Autodesk Fusion 360 part; units mm, degrees
note: some values were not read from the file. Set by a fixed rule: which sketch regions a step uses.
(part 2 of 2)
extrude "Extrude2'''''" cut sketch "End leg - wave" against normal blind 2.54 contours A3 A9 L22 A21 bodies 21 in component "End leg - left (1) (1)"
extrude "Extrude1''''''''''''''''''''" add sketch "Inner leg" along normal blind 18.542 separate body contours L0 L1 L2 A0 A1 L4 L5 A2 L6 A3 L7 L9 L10 L12 A4 A5 L13 L14 L16 A6 A7 L18 L19 L20 L22 L23 L24 A8 A9 A10 A11 L34 L35 L36 L37 L38 L39 L40 A23 A24 L43 L44 L45 A25 makes body 22 in component "Inner leg - right -- middle (1)"
extrude "Extrude1'''''''''''''''''''''" add sketch "Inner leg" along normal blind 18.542 separate body contours L0 L1 L2 A0 A1 L4 L5 A2 L6 A3 L7 L9 L10 L12 A4 A5 L13 L14 L16 A6 A7 L18 L19 L20 L22 L23 L24 A8 A9 A10 A11 L34 L35 L36 L37 L38 L39 L40 A23 A24 L43 L44 L45 A25 makes body 23 in component "Inner leg - right -- left (1)"
extrude "Extrude1''''''''''''''''''''''" add sketch "Inner leg" along normal blind 18.542 separate body contours L0 L1 L2 A0 A1 L4 L5 A2 L6 A3 L7 L9 L10 L12 A4 A5 L13 L14 L16 A6 A7 L18 L19 L20 L22 L23 L24 A8 A9 A10 A11 L34 L35 L36 L37 L38 L39 L40 A23 A24 L43 L44 L45 A25 makes body 24 in component "Inner leg - left -- right (1)"
extrude "Extrude1'''''''''''''''''''''''" add sketch "Inner end leg" along normal blind 18.542 separate body contours A0 L1 L2 L3 A1 L4 A2 A3 A4 A5 L6 L7 L8 L9 A6 A7 L10 L12 A8 L14 A9 L15 L17 L19 L20 L21 L22 A18 L31 L32 L33 L34 L35 L36 L38 L39 L40 L42 A19 A20 makes body 25 in component "Inner leg end (1)"
extrude "Extrude1''''''''''''''''''''''''" add sketch "Inner leg" along normal blind 18.542 separate body contours L0 L1 L2 A0 A1 L4 L5 A2 L6 A3 L7 L9 L10 L12 A4 A5 L13 L14 L16 A6 A7 L18 L19 L20 L22 L23 L24 A8 A9 A10 A11 L34 L35 L36 L37 L38 L39 L40 A23 A24 L43 L44 L45 A25 makes body 26 in component "Inner leg - left -- left (1)"
extrude "Extrude1'''''''''''''''''''''''''" add sketch "Surface" against normal blind 18.542 separate body makes body 27 in component "Surface - right (1)"
extrude "Extrude2''''''" cut sketch "Surface" against normal blind 6.1807 contours L1 L3 L13 L15 | L1 L3 L10 L12 | L1 L3 L7 L9 | L1 L3 A0 L4 L6 bodies 27 in component "Surface - right (1)"
extrude "Extrude1''''''''''''''''''''''''''" add sketch "Spine - long" along normal blind 18.542 separate body contours L0 L3 L4 L5 L7 L8 L9 L11 L12 L13 L14 L15 L16 L21 A0 A1 A2 L27 A6 A7 A8 A9 A10 A11 A12 L30 L31 L32 L33 L34 L39 | L22 L26 L27 L40 | L18 L23 A3 A4 L25 L26 L38 L44 | L19 L24 L25 L46 | L1 L20 A5 L24 A13 L36 L45 | L20 A5 picked at (-72.5108, 47.7756) makes body 28 in component "Long spine (1) (1)"
extrude "Extrude1'''''''''''''''''''''''''''" add sketch "Spine - long" along normal blind 18.542 separate body contours L0 L3 L4 L5 L7 L8 L9 L11 L12 L13 L14 L15 L16 L21 A0 A1 A2 L27 A6 A7 A8 A9 A10 A11 A12 L30 L31 L32 L33 L34 L39 | L22 L26 L27 L40 | L18 L23 A3 A4 L25 L26 L38 L44 | L19 L24 L25 L46 | L1 L20 A5 L24 A13 L36 L45 | L20 A5 picked at (-72.5108, 47.7756) makes body 29 in component "Long spine (1) (2)"
extrude "Extrude1''''''''''''''''''''''''''''" add sketch "Surface" along normal blind 18.542 separate body makes body 30 in component "Surface - left (1)"
extrude "Extrude2'''''''" cut sketch "Surface" along normal blind 6.1807 contours L1 L3 L13 L15 | L1 L3 L10 L12 | L1 L3 L7 L9 | L1 L3 A0 L4 L6 bodies 30 in component "Surface - left (1)"
extrude "Extrude1'''''''''''''''''''''''''''''" add sketch "Spine - short" along normal blind 18.542 separate body contours L0 L1 L3 L4 L5 L6 L7 L8 L10 L11 L12 L14 L15 L16 A0 A1 A2 A3 A4 A5 A6 A7 L17 L18 L19 L20 L21 L22 A8 A9 A10 A11 A12 A13 L23 L24 L26 L27 L29 L30 L32 L33 makes body 31 in component "Short spine (1)"
extrude "Extrude1''''''''''''''''''''''''''''''" add sketch "Spine - short" along normal blind 18.542 separate body contours L0 L1 L3 L4 L5 L6 L7 L8 L10 L11 L12 L14 L15 L16 A0 A1 A2 A3 A4 A5 A6 A7 L17 L18 L19 L20 L21 L22 A8 A9 A10 A11 A12 A13 L23 L24 L26 L27 L29 L30 L32 L33 makes body 32 in component "Short spine (2)"
extrude "Extrude1'''''''''''''''''''''''''''''''" add sketch "Shelf" along normal blind 18.542 separate body contours L0 L1 L2 L3 L4 L5 A0 A1 A2 A3 L8 L9 L10 L12 L13 L14 L15 L16 L17 A4 A5 A6 A7 A8 A9 A10 A11 L18 L19 L20 L22 L23 makes body 33 in component "Shelf - left -- upper (1)"
copy_body "CopyPasteBodies1'" bodies 15 makes body 34 in component "Shelf - left -- lower (1)"
extrude "Extrude1''''''''''''''''''''''''''''''''" add sketch "Shelf" along normal blind 18.542 separate body contours L0 L1 L2 L3 L4 L5 A0 A1 A2 A3 L8 L9 L10 L12 L13 L14 L15 L16 L17 A4 A5 A6 A7 A8 A9 A10 A11 L18 L19 L20 L22 L23 makes body 35 in component "Shelf - right -- lower (1)"
extrude "Extrude1'''''''''''''''''''''''''''''''''" add sketch "Shelf" along normal blind 18.542 separate body contours L0 L1 L2 L3 L4 L5 A0 A1 A2 A3 L8 L9 L10 L12 L13 L14 L15 L16 L17 A4 A5 A6 A7 A8 A9 A10 A11 L18 L19 L20 L22 L23 makes body 36 in component "Shelf - right -- upper (1)"
extrude "Extrude1''''''''''''''''''''''''''''''''''" add sketch "Shelf" along normal blind 18.542 separate body contours L0 L1 L2 L3 L4 L5 A0 A1 A2 A3 L8 L9 L10 L12 L13 L14 L15 L16 L17 A4 A5 A6 A7 A8 A9 A10 A11 L18 L19 L20 L22 L23 makes body 37 in component "Shelf"
sketch "Stock - shelf jig" plane through (0, 0, 0) normal (0, 1, 0) x (1, 0, 0)
  line L0 (0, 0) -> (873.125, 0)
  line L1 (873.125, 0) -> (873.125, 254)
  line L2 (873.125, 254) -> (0, 254)
  line L3 (0, 254) -> (0, 0)
  dimension "d3885" = 873.125
  dimension "d3886" = 254
  measures "d3885" distance of L0.start L0.end
  measures "d3886" distance of L0.start L2.end
extrude "Extrude1'''''''''''''''''''''''''''''''''''" add sketch "Stock - shelf jig" along normal blind 18.542 separate body makes body 38 in component "Stock - shelf"
sketch "Stock - spine (long) jig" plane through (0, 0, 0) normal (0, 1, 0) x (1, 0, 0)
  line L0 (0, 0) -> (1168.4, 0)
  line L1 (1168.4, 0) -> (1168.4, 101.6)
  line L2 (1168.4, 101.6) -> (0, 101.6)
  line L3 (0, 101.6) -> (0, 0)
  line L4 (787.4, 0) -> (787.4, 101.6)
  dimension "d3905" = 101.6
  dimension "d3906" = 1168.4
  dimension "d3938" = 787.4
  measures "d3905" distance of L0.start L2.end
  measures "d3906" distance of L0.start L0.end
  measures "d3938" distance of L3 L4
extrude "Extrude1''''''''''''''''''''''''''''''''''''" add sketch "Stock - spine (long) jig" along normal blind 18.542 separate body contours L0 L2 L3 L4 makes body 39 in component "Stock - spine (long) - bottom"
extrude "Extrude1'''''''''''''''''''''''''''''''''''''" add sketch "Stock - spine (long) jig" along normal blind 18.542 separate body makes body 40 in component "Stock - spine (long) - top"
extrude "Extrude1''''''''''''''''''''''''''''''''''''''" add sketch "Spine - long" along normal blind 18.542 separate body contours L0 L3 L4 L5 L7 L8 L9 L11 L12 L13 L14 L15 L16 L21 A0 A1 A2 L27 A6 A7 A8 A9 A10 A11 A12 L30 L31 L32 L33 L34 L39 | L22 L26 L27 L40 | L18 L23 A3 A4 L25 L26 L38 L44 | L19 L24 L25 L46 | L1 L20 A5 L24 A13 L36 L45 | L20 A5 picked at (-72.5108, 47.7756) makes body 41 in component "Spine (long) - top"
extrude "Extrude1'''''''''''''''''''''''''''''''''''''''" add sketch "Spine - long" along normal blind 18.542 separate body contours L0 L3 L4 L5 L7 L8 L9 L11 L12 L13 L14 L15 L16 L21 A0 A1 A2 L27 A6 A7 A8 A9 A10 A11 A12 L30 L31 L32 L33 L34 L39 | L22 L26 L27 L40 | L18 L23 A3 A4 L25 L26 L38 L44 | L19 L24 L25 L46 | L1 L20 A5 L24 A13 L36 L45 | L20 A5 picked at (-72.5108, 47.7756) makes body 42 in component "Spine (long) - bottom"
sketch "Stock - spine (short) jig" plane through (0, 0, 0) normal (0, 1, 0) x (1, 0, 0)
  line L0 (0, 0) -> (914.4, 0)
  line L1 (914.4, 0) -> (914.4, 101.6)
  line L2 (914.4, 101.6) -> (0, 101.6)
  line L3 (0, 101.6) -> (0, 0)
  dimension "d3943" = 101.6
  dimension "d3944" = 914.4
  measures "d3943" distance of L0.start L2.end
  measures "d3944" distance of L0.start L0.end
extrude "Extrude1''''''''''''''''''''''''''''''''''''''''" add sketch "Stock - spine (short) jig" along normal blind 18.542 separate body makes body 43 in component "Stock - spine (short)"
extrude "Extrude1'''''''''''''''''''''''''''''''''''''''''" add sketch "Spine - short" along normal blind 18.542 separate body contours L0 L1 L3 L4 L5 L6 L7 L8 L10 L11 L12 L14 L15 L16 A0 A1 A2 A3 A4 A5 A6 A7 L17 L18 L19 L20 L21 L22 A8 A9 A10 A11 A12 A13 L23 L24 L26 L27 L29 L30 L32 L33 makes body 44 in component "Spine (short) - top"
extrude "Extrude1''''''''''''''''''''''''''''''''''''''''''" add sketch "Spine - short" along normal blind 18.542 separate body contours L0 L1 L3 L4 L5 L6 L7 L8 L10 L11 L12 L14 L15 L16 A0 A1 A2 A3 A4 A5 A6 A7 L17 L18 L19 L20 L21 L22 A8 A9 A10 A11 A12 A13 L23 L24 L26 L27 L29 L30 L32 L33 makes body 45 in component "Spine (short) - bottom"
extrude "Extrude1'''''''''''''''''''''''''''''''''''''''''''" add sketch "Surface" against normal blind 18.542 separate body makes body 46 in component "Surface for radius operation"
extrude "Extrude2''''''''" cut sketch "Surface" against normal blind 6.1807 contours L1 L3 L13 L15 | L1 L3 L10 L12 | L1 L3 L7 L9 | L1 L3 A0 L4 L6 bodies 46 in component "Surface for radius operation"
sketch "Stock - surface radius jig" plane through (0, 0, 0) normal (0, 1, 0) x (1, 0, 0)
  line L0 (0, 0) -> (76.2, 0)
  line L1 (76.2, 0) -> (76.2, 762)
  line L2 (76.2, 762) -> (0, 762)
  line L3 (0, 762) -> (0, 0)
  dimension "d4039" = 762
  dimension "d4040" = 76.2
  measures "d4039" distance of L0.start L2.end
  measures "d4040" distance of L0.start L0.end
extrude "Extrude1''''''''''''''''''''''''''''''''''''''''''''" add sketch "Stock - surface radius jig" along normal blind 18.542 separate body makes body 47 in component "Stock - surface radius"
extrude "Extrude1'''''''''''''''''''''''''''''''''''''''''''''" add sketch "Surface" against normal blind 18.542 separate body makes body 48 in component "Surface for slot operation"
extrude "Extrude2'''''''''" cut sketch "Surface" against normal blind 6.1807 contours L1 L3 L13 L15 | L1 L3 L10 L12 | L1 L3 L7 L9 | L1 L3 A0 L4 L6 bodies 48 in component "Surface for slot operation"
component "Assembled" placed x (1, 0, 0) y (0, 1, 0) z (0, 0, 1) at (0, 0, 0)
component "Fabrication" placed x (1, 0, 0) y (0, 1, 0) z (0, 0, 1) at (0, 0, 0)
component "Surface - left" placed x (0, 0, -1) y (0, 1, 0) z (1, 0, 0) at (2582.0041, 744.1354, 574.929) in component "Surfaces"
component "Surface - right" placed x (-1, 0, 0) y (0, -1, 0) z (0, 0, 1) at (1820.037, 744.1354, 571.4671) in component "Surfaces"
component "Inner leg - left -- left" placed x (1, 0, 0) y (0, 1, 0) z (0, 0, 1) at (2582.1218, 0.6388, -723.392) in component "Left side"
component "Inner leg - left -- right" placed x (1, 0, 0) y (0, 1, 0) z (0, 0, 1) at (2582.1218, 0.6388, -183.642) in component "Left side"
component "Inner leg end" placed x (1, 0, 0) y (0, 1, 0) z (0, 0, 1) at (2582.037, 0.6388, 356.108) in component "Left side"
component "Inner leg - right -- right" placed x (0, 0, 1) y (0, 1, 0) z (-1, 0, 0) at (540.258, 0, 571.5) in component "Right side"
component "Inner leg - right -- middle" placed x (0, 0, 1) y (0, 1, 0) z (-1, 0, 0) at (1080.008, 0, 571.5) in component "Right side"
component "Inner leg - right -- left" placed x (0, 0, 1) y (0, 1, 0) z (-1, 0, 0) at (1619.758, 0, 571.5) in component "Right side"
component "Left side" placed x (1, 0, 0) y (0, 1, 0) z (0, 0, 1) at (0, 0, 0) in component "Inner legs"
component "Right side" placed x (1, 0, 0) y (0, 1, 0) z (0, 0, 1) at (0, 0, 0) in component "Inner legs"
component "Shelves -- left" placed x (1, 0, 0) y (0, 1, 0) z (0, 0, 1) at (0, 0, 0) in component "Shelves"
component "Shelves -- right" placed x (1, 0, 0) y (0, 1, 0) z (0, 0, 1) at (0, 0, 0) in component "Shelves"
component "Shelf - left -- upper" placed x (1, 0, 0) y (0, 1, 0) z (0, 0, 1) at (2328.037, 420.3954, 428.879) in component "Shelves -- left"
component "Shelf - left -- lower" placed x (1, 0, 0) y (0, 1, 0) z (0, 0, 1) at (2328.037, 115.5954, 428.879) in component "Shelves -- left"
component "Long spines" placed x (1, 0, 0) y (0, 1, 0) z (0, 0, 1) at (0, 0, 0) in component "Spines"
component "Short spines" placed x (1, 0, 0) y (0, 1, 0) z (0, 0, 1) at (0, 0, 0) in component "Spines"
component "Long spine (1)" placed x (1, 0, 0) y (0, 1, 0) z (0, 0, 1) at (2366.137, 641.731, 98.679) in component "Long spines"
component "Long spine (1)" placed x (1, 0, 0) y (0, 1, 0) z (0, 0, 1) at (2366.137, 642.4968, 263.779) in component "Long spines"
component "Short spine" placed x (1, 0, 0) y (0, 1, 0) z (0, 0, 1) at (2109.216, 642.4968, 511.429) in component "Short spines"
component "Short spine" placed x (1, 0, 0) y (0, 1, 0) z (0, 0, 1) at (2274.316, 642.4968, 511.429) in component "Short spines"
component "End leg - right (1)" placed x (1, 0, 0) y (0, 1, 0) z (0, 0, 1) at (-18.034, 0, 0) in component "End legs"
component "End leg - left (1)" placed x (0, 0, -1) y (0, 1, 0) z (1, 0, 0) at (2010.537, 0, -1263.142) in component "End legs"
component "Surfaces" placed x (1, 0, 0) y (0, 1, 0) z (0, 0, 1) at (0, 0, 0) in component "Assembled"
component "Inner legs" placed x (1, 0, 0) y (0, 1, 0) z (0, 0, 1) at (0, 0, 0) in component "Assembled"
component "Shelves" placed x (1, 0, 0) y (0, 1, 0) z (0, 0, 1) at (0, 0, 0) in component "Assembled"
component "Spines" placed x (1, 0, 0) y (0, 1, 0) z (0, 0, 1) at (0, 0, 0) in component "Assembled"
component "End legs" placed x (1, 0, 0) y (0, 1, 0) z (0, 0, 1) at (0, 0, 0) in component "Assembled"
component "Stock - 4x8'" placed x (1, 0, 0) y (0, 1, 0) z (0, 0, 1) at (0, 0, 0) in component "Fabrication"
component "Stock - 4x4'" placed x (1, 0, 0) y (0, 1, 0) z (0, 0, 1) at (0, 0, 0) in component "Fabrication"
component "Sheet 1 - end leg (right) + inner leg x1" placed x (1, 0, 0) y (0, 1, 0) z (0, 0, 1) at (0, 0, 0) in component "Fabrication"
component "Sheet 2 - end leg (left) + inner leg x1" placed x (1, 0, 0) y (0, 1, 0) z (0, 0, 1) at (0, 0, 0) in component "Fabrication"
component "Sheet 3 - inner leg x2" placed x (1, 0, 0) y (0, 1, 0) z (0, 0, 1) at (0, 0, 0) in component "Fabrication"
component "Sheet 4 - inner end leg + inner leg x1" placed x (1, 0, 0) y (0, 1, 0) z (0, 0, 1) at (0, 0, 0) in component "Fabrication"
component "Sheet 5 - surface (right) + long spines" placed x (1, 0, 0) y (0, 1, 0) z (0, 0, 1) at (0, 0, 0) in component "Fabrication"
component "Sheet 6 - surface (left) + short spines" placed x (1, 0, 0) y (0, 1, 0) z (0, 0, 1) at (0, 0, 0) in component "Fabrication"
component "Sheet 7 - shelves" placed x (1, 0, 0) y (0, 1, 0) z (0, 0, 1) at (0, 0, 0) in component "Fabrication"
component "Jig - shelf" placed x (1, 0, 0) y (0, 1, 0) z (0, 0, 1) at (0, 0, 0) in component "Fabrication"
component "Jigs - long spine" placed x (1, 0, 0) y (0, 1, 0) z (0, 0, 1) at (0, 0, 0) in component "Fabrication"
component "Jigs - short spine" placed x (1, 0, 0) y (0, 1, 0) z (0, 0, 1) at (0, 0, 0) in component "Fabrication"
component "Jigs - surface radius and slot" placed x (1, 0, 0) y (0, 1, 0) z (0, 0, 1) at (0, 0, 0) in component "Fabrication"
component "Shelf - right -- lower" placed x (0, 0, 1) y (0, 1, 0) z (-1, 0, 0) at (-72.263, 115.5954, 317.5) in component "Shelves -- right"
component "Shelf - right -- upper" placed x (0, 0, 1) y (0, 1, 0) z (-1, 0, 0) at (-72.263, 420.3954, 317.5) in component "Shelves -- right"
component "End leg - right (1) (1)" placed x (0, -1, 0) y (1, 0, 0) z (0, 0, 1) at (408.533, 18.542, 520.0921) in component "Sheet 1 - end leg (right) + inner leg x1"
component "Inner leg - right -- right (1)" placed x (-1, 0, 0) y (0, 0, -1) z (0, -1, 0) at (78.8, 18.542, 990.0892) in component "Sheet 1 - end leg (right) + inner leg x1"
component "End leg - left (1) (1)" placed x (0, 1, 0) y (0, 0, 1) z (1, 0, 0) at (296.1006, 18.542, 127.0302) in component "Sheet 2 - end leg (left) + inner leg x1"
component "Inner leg - right -- middle (1)" placed x (-1, 0, 0) y (0, 0, -1) z (0, -1, 0) at (454.1371, 18.542, 1099.058) in component "Sheet 2 - end leg (left) + inner leg x1"
component "Inner leg - right -- left (1)" placed x (-1, 0, 0) y (0, 0, -1) z (0, -1, 0) at (454.1371, 18.542, 1099.058) in component "Sheet 3 - inner leg x2"
component "Inner leg - left -- right (1)" placed x (1, 0, 0) y (0, 0, 1) z (0, -1, 0) at (765.0629, 18.542, 120.142) in component "Sheet 3 - inner leg x2"
component "Inner leg end (1)" placed x (0, 0, -1) y (1, 0, 0) z (0, -1, 0) at (107.442, 18.542, 274.1395) in component "Sheet 4 - inner end leg + inner leg x1"
component "Inner leg - left -- left (1)" placed x (1, 0, 0) y (0, 0, 1) z (0, -1, 0) at (765.0629, 18.542, 120.142) in component "Sheet 4 - inner end leg + inner leg x1"
component "Surface - right (1)" placed x (1, 0, 0) y (0, 1, 0) z (0, 0, 1) at (266.7, 18.542, 990.6) in component "Sheet 5 - surface (right) + long spines"
component "Long spine (1) (1)" placed x (1, 0, 0) y (0, 0, 1) z (0, -1, 0) at (2438.4, 18.542, 558.8) in component "Sheet 5 - surface (right) + long spines"
component "Long spine (1) (2)" placed x (1, 0, 0) y (0, 0, 1) z (0, -1, 0) at (2438.4, 18.542, 558.8) in component "Sheet 5 - surface (right) + long spines"
component "Surface - left (1)" placed x (1, 0, 0) y (0, -1, 0) z (0, 0, -1) at (266.7, 18.542, 228.6) in component "Sheet 6 - surface (left) + short spines"
component "Short spine (1)" placed x (0, 1, 0) y (0, 0, 1) z (1, 0, 0) at (2133.6, 0, 558.8) in component "Sheet 6 - surface (left) + short spines"
component "Short spine (2)" placed x (0, 1, 0) y (0, 0, 1) z (1, 0, 0) at (2133.6, 0, 558.8) in component "Sheet 6 - surface (left) + short spines"
component "Shelf - left -- upper (1)" placed x (0, 0, -1) y (0, -1, 0) z (-1, 0, 0) at (346.075, 18.542, 736.6) in component "Sheet 7 - shelves"
component "Shelf - left -- lower (1)" placed x (0, 0, -1) y (0, -1, 0) z (-1, 0, 0) at (346.075, 18.542, 736.6) in component "Sheet 7 - shelves"
component "Shelf - right -- lower (1)" placed x (0, 0, 1) y (0, -1, 0) z (1, 0, 0) at (2092.325, 18.542, 482.6) in component "Sheet 7 - shelves"
component "Shelf - right -- upper (1)" placed x (0, 0, 1) y (0, -1, 0) z (1, 0, 0) at (2092.325, 18.542, 482.6) in component "Sheet 7 - shelves"
component "Shelf" placed x (0, 0, 1) y (0, 1, 0) z (-1, 0, 0) at (-873.125, 0, -254) in component "Jig - shelf"
component "Stock - shelf" placed x (1, 0, 0) y (0, 1, 0) z (0, 0, 1) at (0, 0, 0) in component "Jig - shelf"
component "Stock - spine (long) - top" placed x (1, 0, 0) y (0, 1, 0) z (0, 0, 1) at (0, 0, 0) in component "Jigs - long spine"
component "Spine (long) - top" placed x (-1, 0, 0) y (0, 0, 1) z (0, 1, 0) at (-1270, 0, -101.6) in component "Jigs - long spine"
component "Spine (long) - bottom" placed x (1, 0, 0) y (0, 0, 1) z (0, -1, 0) at (787.4, 18.542, -101.6) in component "Jigs - long spine"
component "Stock - spine (long) - bottom" placed x (1, 0, 0) y (0, 1, 0) z (0, 0, 1) at (0, 0, 0) in component "Jigs - long spine"
component "Stock - spine (short)" placed x (1, 0, 0) y (0, 1, 0) z (0, 0, 1) at (0, 0, 0) in component "Jigs - short spine"
component "Spine (short) - top" placed x (0, 1, 0) y (0, 0, 1) z (1, 0, 0) at (914.4, 0, -101.6) in component "Jigs - short spine"
component "Spine (short) - bottom" placed x (0, -1, 0) y (0, 0, 1) z (-1, 0, 0) at (-914.4, 18.542, -101.6) in component "Jigs - short spine"
component "Surface for radius operation" placed x (1, 0, 0) y (0, 1, 0) z (0, 0, 1) at (-1828.8, 18.542, 0) in component "Jigs - surface radius and slot"
component "Stock - surface radius" placed x (1, 0, 0) y (0, 1, 0) z (0, 0, 1) at (0, 0, 0) in component "Jigs - surface radius and slot"
component "Surface for slot operation" placed x (1, 0, 0) y (0, 1, 0) z (0, 0, 1) at (-199.009, 18.542, 762) in component "Jigs - surface radius and slot"
equation "d2 = Depth"
equation "Depth = 30 in"
equation "Thickness_Surface = Thickness_Global"
equation "SegmentLength = 72 in"
equation "Thickness_Legs = Thickness_Global"
equation "Fit_Interference = ( 0.011 * 2 ) * 1 in"
equation "Fit_Clearance = 0.1 in"
equation "d25 = Bench_Height - Thickness_Surface"
equation "Bench_Height = 30 in"
equation "d27 = Depth * 0.75"
equation "Depth_Engrave = 0.1 in"
equation "d38 = d37"
equation "d41 = Thickness_Legs"
equation "Bolt_Diameter = 8 mm"
equation "d45 = 21.25 in"
equation "d46 = d45"
equation "d48 = d52 / 2"
equation "d49 = d48"
equation "d50 = d49"
equation "d52 = d2 / 2"
equation "d54 = d52"
equation "d55 = d54"
equation "d103 = Depth / 3"
equation "d41_1 = Thickness_Legs"
equation "d41_2 = Thickness_Legs"
equation "d41_2_1 = Thickness_Legs"
equation "d41_2_2 = Thickness_Legs"
equation "d121 = d2 / 2"
equation "d122 = d121"
equation "Lower_Shelf_Height = Bench_Height / 5 - Thickness_Legs"
equation "d129 = End_Mill_Diameter"
equation "End_Mill_Diameter = 0.25 in"
equation "d133 = Shelf_Support_Thickness + Fit_Clearance"
equation "d136 = Shelf_Support_Height / 2"
equation "d137 = Lower_Shelf_Height"
equation "d138 = d103 / 5"
equation "Shelf_Support_Height = 2.5 in"
equation "d151 = d136"
equation "d152 = d138"
equation "d153 = Upper_Shelf_Height"
equation "Upper_Shelf_Height = Bench_Height / 5 * 3 - Thickness_Legs"
equation "d162 = d171"
equation "d171 = Shelf_Support_Thickness + Fit_Clearance"
equation "d176 = d162"
equation "d182 = End_Mill_Diameter"
equation "d183 = End_Mill_Diameter"
equation "Shelf_Support_Thickness = Thickness_Global"
equation "d249 = Lower_Shelf_Height"
equation "Shelf_Support_Length = ( 4 * 12 ) * 1 in"
equation "d270 = d46"
equation "d277 = d270"
equation "d280 = d277 / 2"
equation "d283 = d50"
equation "d286 = d50"
equation "d289 = d286"
equation "Shelf_Depth = 10 in"
equation "d314 = Thickness_Shelf - Fit_Interference"
equation "d316 = End_Mill_Diameter"
equation "d317 = End_Mill_Diameter"
equation "Thickness_Shelf = Thickness_Legs"
equation "d320 = d314"
equation "d322 = End_Mill_Diameter"
equation "d323 = End_Mill_Diameter"
equation "d328 = Shelf_Depth / 2"
equation "d329 = End_Mill_Diameter"
equation "d330 = End_Mill_Diameter"
equation "d331 = Thickness_Shelf - Fit_Interference"
equation "d332 = Upper_Shelf_Height"
equation "d333 = d328"
equation "d334 = d331"
equation "d335 = End_Mill_Diameter"
equation "d336 = End_Mill_Diameter"
equation "d337 = Lower_Shelf_Height"
equation "d382 = Cable_Channel_Width"
equation "d385 = Cable_Channel_Width"
equation "Tab_Size = 2 in"
equation "d466 = Depth / 2 / 2"
equation "d493 = Shelf_Depth / 2"
equation "d494 = Thickness_Legs - Fit_Interference"
equation "d497 = d496"
equation "d498 = d499"
equation "d499 = d497"
equation "d500 = d493"
equation "d501 = d494"
equation "d503 = d501"
equation "d504 = d500"
equation "d505 = d502"
equation "d506 = d504"
equation "d507 = d503"
equation "d508 = d505"
equation "d509 = End_Mill_Diameter"
equation "d510 = End_Mill_Diameter"
equation "d511 = End_Mill_Diameter"
equation "d512 = End_Mill_Diameter"
equation "d513 = End_Mill_Diameter"
equation "d514 = End_Mill_Diameter"
equation "d515 = End_Mill_Diameter"
equation "d516 = End_Mill_Diameter"
equation "Spine_Height = 4 in"
equation "d772 = Thickness_Legs - Fit_Interference"
equation "d773 = Spine_Height / 2"
equation "d774 = d772"
equation "d775 = Spine_Height / 2"
equation "d776 = End_Mill_Diameter"
equation "d777 = End_Mill_Diameter"
equation "d778 = End_Mill_Diameter"
equation "d779 = End_Mill_Diameter"
equation "d781 = 13.00 in / 2"
equation "d782 = d781 / 2"
equation "d783 = d782"
equation "d834 = Spine_Height"
equation "d835 = Thickness_Legs"
equation "d839 = Thickness_Legs - Fit_Interference"
equation "d840 = Spine_Height / 2"
equation "d841 = d839"
equation "d842 = d840"
equation "d843 = d842"
equation "d844 = d841"
equation "d845 = d846"
equation "d848 = d844"
equation "d849 = d843"
equation "d850 = d853"
equation "d851 = d852"
equation "d852 = d849"
equation "d853 = d848"
equation "d854 = d845"
equation "d857 = End_Mill_Diameter"
equation "d858 = End_Mill_Diameter"
equation "d859 = End_Mill_Diameter"
equation "d860 = End_Mill_Diameter"
equation "d861 = End_Mill_Diameter"
equation "d862 = End_Mill_Diameter"
equation "d863 = End_Mill_Diameter"
equation "d864 = End_Mill_Diameter"
equation "d865 = End_Mill_Diameter"
equation "d866 = End_Mill_Diameter"
equation "d867 = End_Mill_Diameter"
equation "d868 = End_Mill_Diameter"
equation "d869 = Thickness_Legs - Fit_Interference"
equation "d870 = Spine_Height / 2"
equation "d871 = d869"
equation "d872 = d870"
equation "d875 = 13.00 in / 2"
equation "d876 = d875 / 2"
equation "d877 = d876"
equation "d878 = End_Mill_Diameter"
equation "d879 = End_Mill_Diameter"
equation "d880 = End_Mill_Diameter"
equation "d881 = End_Mill_Diameter"
equation "d906 = 6'-0\""
equation "d907 = Spine_Height"
equation "d908 = Thickness_Legs - Fit_Interference"
equation "d909 = Spine_Height / 2"
equation "d912 = d908"
equation "d913 = d909"
equation "d914 = d912"
equation "d915 = d913"
equation "d916 = d969"
equation "d917 = d970"
equation "d926 = Thickness_Legs"
equation "d928 = End_Mill_Diameter"
equation "d929 = End_Mill_Diameter"
equation "d930 = End_Mill_Diameter"
equation "d931 = End_Mill_Diameter"
equation "d932 = End_Mill_Diameter"
equation "d933 = End_Mill_Diameter"
equation "d934 = End_Mill_Diameter"
equation "d935 = End_Mill_Diameter"
equation "d969 = d1382"
equation "d970 = d972"
equation "d972 = d915"
equation "d973 = End_Mill_Diameter"
equation "d974 = End_Mill_Diameter"
equation "d975 = End_Mill_Diameter"
equation "d976 = End_Mill_Diameter"
equation "d977 = 4 in - Thickness_Legs / 2"
equation "d982 = Spine_Height / 2"
equation "d983 = Spine_Height / 2"
equation "d984 = Spine_Height / 2"
equation "d985 = Spine_Height / 2"
equation "d987 = Shelf_Depth / 2"
equation "d1017 = Thickness_Shelf - Fit_Interference"
equation "d1019 = End_Mill_Diameter"
equation "d1020 = End_Mill_Diameter"
equation "d1021 = d1017"
equation "d1023 = End_Mill_Diameter"
equation "d1024 = End_Mill_Diameter"
equation "d1025 = d314 / 2"
equation "d1026 = d320 / 2"
equation "d1033 = Thickness_Legs - Fit_Interference"
equation "d1034 = Spine_Height / 2"
equation "d1036 = d1034"
equation "d1037 = End_Mill_Diameter"
equation "d1038 = End_Mill_Diameter"
equation "d1039 = End_Mill_Diameter"
equation "d1040 = End_Mill_Diameter"
equation "d1042 = d781 / 2"
equation "d1043 = d782"
equation "d1062 = Lower_Shelf_Height"
equation "d1063 = Upper_Shelf_Height"
equation "d1064 = Thickness_Legs"
equation "d1107 = d1106"
equation "d1108 = d1105"
equation "d1109 = d1104"
equation "d1110 = d1109"
equation "d1382 = d914"
equation "d2574 = d2571"
equation "d2577 = d2571"
equation "d2653 = 3 in"
equation "d2663 = d2653"
equation "d2674 = d2663"
equation "Thickness_Global = 0.73 in"
equation "d2750 = End_Mill_Diameter"
equation "d2751 = End_Mill_Diameter"
equation "d2754 = Thickness_Global"
equation "Leg_Spacing = 21.25 in"
equation "d2962 = Shelf_Depth / 2"
equation "d2964 = d1250"
equation "d2965 = Shelf_Depth / 2"
equation "d2969 = Thickness_Surface / 3"
equation "d2970 = Thickness_Surface / 3"
equation "d2972 = Bench_Height - Thickness_Surface + Thickness_Surface / 3"
equation "d2974 = Thickness_Legs - Fit_Interference"
equation "d2975 = d2974"
equation "d2976 = d1062"
equation "Cable_Channel_Width = 0.5 in"
equation "d2980 = Thickness_Surface / 3"
equation "d2981 = Depth"
equation "d3009 = Thickness_Legs"
equation "d3011 = Depth_Engrave"
equation "d3013 = -Thickness_Legs"
equation "d3015 = -Depth_Engrave"
equation "d3017 = Shelf_Depth"
equation "d3022 = Shelf_Depth / 2"
equation "d3024 = Bench_Height - Thickness_Surface + Thickness_Surface / 3"
equation "d3025 = Lower_Shelf_Height"
equation "d3027 = Upper_Shelf_Height"
equation "d3028 = Shelf_Depth / 2"
equation "d3030 = d3036"
equation "d3032 = Thickness_Surface / 3"
equation "d3034 = d3032"
equation "d3036 = Cable_Channel_Width / 2"
equation "d3039 = Surface_Length"
equation "d3040 = Depth"
equation "d3041 = Surface_Radius"
equation "d3042 = ( Thickness_Legs / 2 ) + Fit_Clearance / 2"
equation "d3043 = d3042"
equation "d3045 = d3042"
equation "d3046 = d3045"
equation "d3047 = Leg_Spacing"
equation "d3048 = d3046"
equation "d3049 = d3048"
equation "d3050 = d3049"
equation "d3051 = d3049"
equation "d3052 = d3047"
equation "d3053 = d3052"
equation "d3054 = Thickness_Surface"
equation "d3056 = Thickness_Surface / 3"
equation "d3058 = -Thickness_Surface"
equation "d3060 = -Thickness_Surface / 3"
equation "d3290 = Thickness_Shelf"
equation "d3290_1 = Thickness_Shelf"
equation "Surface_Length = 105 in - Depth"
equation "d3290_2 = Thickness_Shelf"
equation "d3389 = Leg_Spacing"
equation "d3401 = -Leg_Spacing"
equation "d3413 = -Leg_Spacing"
equation "d3592 = d980"
equation "d3599 = Thickness_Global"
equation "d3009_1 = Thickness_Legs"
equation "d3011_1 = Depth_Engrave"
equation "d3612 = -Thickness_Global"
equation "d41_2_3 = Thickness_Legs"
equation "d3624 = -Thickness_Global"
equation "d3013_1 = -Thickness_Legs"
equation "d3015_1 = -Depth_Engrave"
equation "d3652 = -Thickness_Global"
equation "d41_2_1_1 = Thickness_Legs"
equation "d3664 = -Thickness_Global"
equation "d41_2_2_1 = Thickness_Legs"
equation "d3684 = -Thickness_Global"
equation "d41_1_1 = Thickness_Legs"
equation "d1064_1 = Thickness_Legs"
equation "d41_3 = Thickness_Legs"
equation "d3058_1 = -Thickness_Surface"
equation "d3060_1 = -Thickness_Surface / 3"
equation "d3748 = -Thickness_Global"
equation "d835_1 = Thickness_Legs"
equation "d835_2 = Thickness_Legs"
equation "d3054_1 = Thickness_Surface"
equation "d3056_1 = Thickness_Surface / 3"
equation "d3792 = -Thickness_Global"
equation "d926_1 = Thickness_Legs"
equation "d3804 = -Thickness_Global"
equation "d926_2 = Thickness_Legs"
equation "d3816 = -Thickness_Global"
equation "d3290_2_1 = Thickness_Shelf"
equation "d3828 = -Thickness_Global"
equation "d3840 = -Thickness_Global"
equation "d3290_1_1 = Thickness_Shelf"
equation "d3852 = -Thickness_Global"
equation "d3290_3 = Thickness_Shelf"
equation "d3864 = -Thickness_Global"
equation "d3290_2_1_1 = Thickness_Shelf"
equation "d3886 = Shelf_Depth"
equation "d3887 = Thickness_Global"
equation "d3900 = -Thickness_Shelf"
equation "d3905 = Spine_Height"
equation "d3909 = Thickness_Global"
equation "d835_1_1 = Thickness_Legs"
equation "d835_1_1_1 = Thickness_Legs"
equation "d3936 = Thickness_Global"
equation "d3943 = Spine_Height"
equation "d3945 = Thickness_Global"
equation "d926_1_1 = Thickness_Legs"
equation "d926_1_1_1 = Thickness_Legs"
equation "d4006 = -Thickness_Global"
equation "d3058_1_1 = -Thickness_Surface"
equation "d3060_1_1 = -Thickness_Surface / 3"
equation "d4039 = Depth"
equation "d4040 = Surface_Radius"
equation "Surface_Radius = 3 in"
equation "d4042 = Thickness_Global"
equation "d3058_1_1_1 = -Thickness_Surface"
equation "d3060_1_1_1 = -Thickness_Surface / 3"
